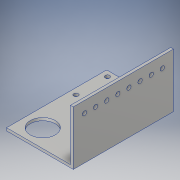
# Autodesk Inventor part: ARM_067_NewLongShaftMount
Saved by Autodesk Inventor 2018 (Build 220112000, 112)
## iProperties
Created: 2020-02-11
Part Number: ARM_067_NewLongShaftMount
Material: Aluminum 6061
Document SubType Name: Modeling
Designer: user
Mass: 129.97 g
Surface Area: 319.153 cm^2
Volume: 48.137 cm^3
Density: 2.7 g/cm^3
Appearance: Aluminum - Flat
Author: user
Autodesk Inventor part; units mm, degrees
ref_plane "YZ Plane" through (0, 0, 0) normal (1, 0, 0) x (0, 1, 0)
ref_plane "XZ Plane" through (0, 0, 0) normal (0, 1, 0) x (-1, 0, 0)
ref_plane "XY Plane" through (0, 0, 0) normal (0, 0, 1) x (1, 0, 0)
sketch "Sketch1" plane through (0, 0, 0) normal (0, 0, 1) x (1, 0, 0)
  line L0 (0, 0) -> (76.2, 0)
  line L1 (76.2, 0) -> (76.2, 76.2)
  line L2 (76.2, 76.2) -> (0, 76.2)
  line L3 (0, 3.175) -> (0, 0)
  line L4 (3.175, 3.175) -> (73.025, 3.175)
  line L5 (73.025, 3.175) -> (73.025, 73.025)
  line L6 (3.175, 3.175) -> (0, 3.175)
  line L7 (73.025, 73.025) -> (73.025, 76.2)
  dimension "d0" = 76.2
  dimension "d1" = 76.2
  constraints: 16 end point, 2 horizontal, 2 parallel, 2 perpendicular, 1 point on line, 1 vertical, 1 other
  measures "d0" distance of L2.end L1.end
  measures "d1" distance of L1.end L0.end
extrude "Extrusion1" add sketch "Sketch1" along normal blind 114.3
sketch "Sketch2" plane through (0, 0, 0) normal (0, -1, 0) x (1, 0, 0)
  line L0 (0, 114.3) -> (76.2, 114.3) projected
  line L1 (0, 0) -> (0, 114.3) projected
  point P0 (20.6375, 93.6625)
  dimension "d5" = 20.6375
  dimension "d6" = 20.6375
  dimension "d14" = 114.3
  measures "d5" distance from line of L0 point (20.637, 93.663)
  measures "d6" distance from line of L1 point (20.637, 93.663)
  measures "d14" distance of L1.start L0.start
hole "Hole1" at (20.6375, 0, 93.6625) direction (0, 1, 0) diameter 28.575 depth 25.4 tip angle 118
sketch "Sketch3" plane through (0, 3.175, 0) normal (0, 1, 0) x (1, 0, 0)
  circle A0 centre (20.6375, -93.6625) radius 14.2875 projected
  line L0 (0, 0) -> (0, -114.3) projected
  line L1 (47.625, 18.9706) -> (73.025, 18.9706) construction
  line L2 (73.025, 18.9706) -> (73.025, -101.6) construction
  line L3 (73.025, -101.6) -> (47.625, -101.6) construction
  line L4 (47.625, -101.6) -> (47.625, 18.9706) construction
  line L5 (73.025, 0) -> (73.025, -114.3) construction
  circle A1 centre (25.0952, -24.2603) radius 17.4498 construction
  dimension "d27" = 69.5452
  dimension "d28" = 25.4
  dimension "d29" = 34.8996
  dimension "d30" = 22.5298
  constraints: 8 end point, 2 parallel, 1 centre point, 1 coincident, 1 collinear, 1 horizontal, 1 perpendicular
  measures "d27" distance of point (25.095, -24.26) A0.centre
  measures "d28" distance of L1.start L1.end
  measures "d29" diameter of A1
  measures "d30" distance from line of L4 A1.centre
hole "Hole2" at (25.0952, 3.175, 24.2603) direction (0, -1, 0) diameter 19.05 depth 25.4 tip angle 118
sketch "Sketch4" plane through (0, 3.175, 0) normal (0, 1, 0) x (1, 0, 0)
  line L0 (0, 0) -> (0, -114.3) projected
  circle A0 centre (25.0952, -24.2603) radius 25.4
  line L1 (-11.821, -6.2998) -> (92.2522, -6.2998) construction
  circle A1 centre (25.0952, -24.2603) radius 7.9375
  circle A2 centre (25.0952, -24.2603) radius 9.525 projected
  point P0 (7.1347, -6.2998)
  point P1 (7.1347, -42.2208)
  point P2 (43.0557, -42.2208)
  point P3 (43.0557, -6.2998)
  dimension "d39" = 50.8
  dimension "d42" = 360
  constraints: 2 end point, 2 point on line, 1 centre point, 1 coincident, 1 horizontal, 9 other
hole "Hole3" at (7.1347, 3.175, 6.2998) at (43.0557, 3.175, 6.2998) at (43.0557, 3.175, 42.2208) at (7.1347, 3.175, 42.2208) direction (0, -1, 0) diameter 5.1054 depth 25.4 tip angle 118 clearance for "Flat Head Machine Screw (82)" size "#10" standard "Ansi Unified Screw Threads"
sketch "Sketch5" plane through (0, 0, 0) normal (0, 0, -1) x (-1, 0, 0)
  line L0 (-47.7073, 61.8998) -> (-105.1568, 61.8998)
  line L1 (-105.1568, 61.8998) -> (-105.1568, 87.3508)
  line L2 (-105.1568, 87.3508) -> (-47.7073, 87.3508)
  line L3 (-47.7073, 87.3508) -> (-47.7073, 61.8998)
  line L4 (-76.2, 76.2) -> (-73.025, 76.2) projected
  point P0 (0, 0)
  dimension "d44" = 14.3002
  constraints: 8 end point, 2 parallel, 1 horizontal, 1 perpendicular
  measures "d44" distance between parallel lines of L4 L0
extrude "Extrusion2" cut sketch "Sketch5" against normal through all
sketch "Sketch6" plane through (73.025, 3.175, 0) normal (-1, 0, 0) x (0, 0, 1)
  line L0 (114.3, 58.7248) -> (0, 58.7248) projected
  line L1 (114.3, 58.7248) -> (114.3, 0) projected
  line L2 (0, 58.7248) -> (0, 0) projected
  point P0 (0, -3.175)
  point P1 (101.6, 46.0248)
  point P2 (88.9, 46.0248)
  point P3 (76.2, 46.0248)
  point P4 (63.5, 46.0248)
  point P5 (50.8, 46.0248)
  point P6 (38.1, 46.0248)
  point P7 (25.4, 46.0248)
  point P8 (12.7, 46.0248)
  dimension "d47" = 12.7
  dimension "d48" = 12.7
  dimension "d49" = 12.7
  dimension "d50" = 12.7
  dimension "d51" = 12.7
  dimension "d52" = 12.7
  dimension "d53" = 12.7
  dimension "d54" = 12.7
  dimension "d55" = 12.7
  dimension "d56" = 12.7
  dimension "d57" = 12.7
  dimension "d58" = 12.7
  dimension "d59" = 12.7
  dimension "d60" = 12.7
  dimension "d61" = 12.7
  dimension "d62" = 12.7
  measures "d47" distance from line of L0 point (101.6, 46.025)
  measures "d48" distance from line of point (101.6, 46.025) L1
  measures "d49" distance of point (101.6, 46.025) point (88.9, 46.025)
  measures "d50" distance of point (88.9, 46.025) point (76.2, 46.025)
  measures "d51" distance of point (76.2, 46.025) point (63.5, 46.025)
  measures "d52" distance of point (63.5, 46.025) point (50.8, 46.025)
  measures "d53" distance of point (50.8, 46.025) point (38.1, 46.025)
  measures "d54" distance of point (25.4, 46.025) point (38.1, 46.025)
  measures "d55" distance of point (25.4, 46.025) point (12.7, 46.025)
  measures "d56" distance from line of L2 point (12.7, 46.025)
  measures "d57" distance from line of L0 point (88.9, 46.025)
  measures "d58" distance from line of L0 point (76.2, 46.025)
  measures "d59" distance from line of L0 point (63.5, 46.025)
  measures "d60" distance from line of L0 point (50.8, 46.025)
  measures "d61" distance from line of L0 point (38.1, 46.025)
  measures "d62" distance from line of L0 point (12.7, 46.025)
hole "Hole4" at (73.025, 49.1998, 101.6) at (73.025, 49.1998, 88.9) at (73.025, 49.1998, 76.2) at (73.025, 49.1998, 63.5) at (73.025, 49.1998, 50.8) at (73.025, 49.1998, 38.1) at (73.025, 49.1998, 25.4) at (73.025, 49.1998, 12.7) direction (1, 0, 0) diameter 4.8514 end through all
equation "\"d5\" = d6"
body "Solid1"
